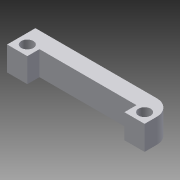
# Autodesk Inventor part: yCarMid_b
Saved by Autodesk Inventor 2013 (Build 170138000, 138)
## iProperties
Created: 2015-01-14
Part Number: yCarMid_b
Material: Generic
Document SubType Name: Modeling
Designer: dzban
Density: 1 g/cm^3
Author: dzban
Autodesk Inventor part; units mm, degrees
ref_plane "YZ Plane" through (0, 0, 0) normal (1, 0, 0) x (0, 1, 0)
ref_plane "XZ Plane" through (0, 0, 0) normal (0, 1, 0) x (-1, 0, 0)
ref_plane "XY Plane" through (0, 0, 0) normal (0, 0, 1) x (1, 0, 0)
sketch "Sketch1" plane through (0, 0, 0) normal (0, 0, 1) x (1, 0, 0)
  circle A0 centre (0, 39) radius 1.5
  circle A1 centre (29, 39) radius 1.5
  line L0 (-2.5, 36.5) -> (2.5, 36.5)
  line L1 (2.5, 36.5) -> (2.5, 39.5)
  line L2 (2.5, 39.5) -> (26.5, 39.5)
  line L3 (26.5, 39.5) -> (26.5, 36.5)
  line L4 (26.5, 36.5) -> (31.5, 36.5)
  line L5 (31.5, 36.5) -> (31.5, 39.5)
  arc A2 (31.5, 39.5) -> (27.5, 43.5) centre (27.5, 39.5) ccw
  line L6 (27.5, 43.5) -> (-2.5, 43.5)
  line L7 (-2.5, 43.5) -> (-2.5, 36.5)
  point P0 (0, 0)
  constraints: 16 end point, 3 centre point, 2 point on circle
extrude "Extrusion1" add sketch "Sketch1" along normal blind 6
body "Solid1"
